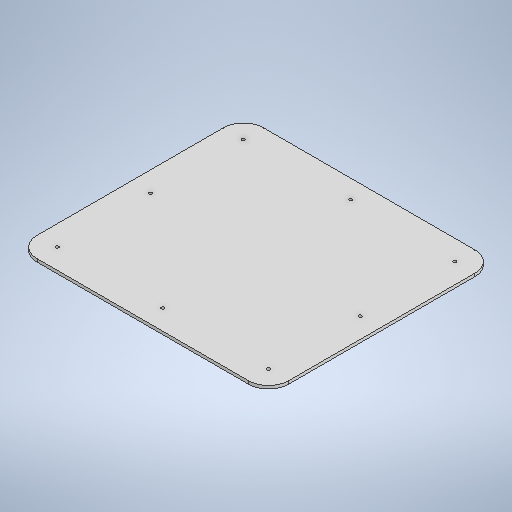
# Autodesk Inventor part: Chassis Top Plate
Saved by Autodesk Inventor 2025.2 (Build 292293000, 293)
## iProperties
Created: 2025-01-24
Part Number: Chassis Top Plate
Material: Generic
Document SubType Name: Modeling
Designer: Matt Tidd
Density: 1 g/cm^3
Appearance: Default
Author: Matt Tidd
Autodesk Inventor part; units mm, degrees
ref_plane "YZ Plane" through (0, 0, 0) normal (1, 0, 0) x (0, 1, 0)
ref_plane "XZ Plane" through (0, 0, 0) normal (0, 1, 0) x (-1, 0, 0)
ref_plane "XY Plane" through (0, 0, 0) normal (0, 0, 1) x (1, 0, 0)
sketch "Sketch2" plane through (0, 0, 0) normal (0, 1, 0) x (-1, 0, 0)
  line L0 (0, 0) -> (250, 0)
  line L1 (250, 0) -> (250, -125)
  line L2 (0, -125) -> (0, 0)
  line L3 (125, 0) -> (125, -125) construction
  line L4 (125, -125) -> (200, -125)
  line L5 (200, -125) -> (200, -225)
  line L6 (200, -225) -> (125, -225)
  line L7 (125, -225) -> (125, -125) construction
  line L8 (125, -125) -> (50, -125)
  line L9 (50, -125) -> (50, -225)
  line L10 (50, -225) -> (125, -225)
  line L11 (125, -225) -> (125, -125) construction
  line L12 (200, -125) -> (250, -125)
  line L13 (0, -125) -> (50, -125)
  line L14 (250, 0) -> (0, 0)
  line L15 (0, 0) -> (0, -225)
  line L16 (0, -225) -> (250, -225)
  line L17 (250, -225) -> (250, 0)
  dimension "d36" = 250
  dimension "d37" = 125
  dimension "d38" = 75
  dimension "d39" = 100
  dimension "d40" = 75
  dimension "d41" = 100
  constraints: 36 end point, 8 equal length, 5 horizontal, 4 perpendicular, 1 midpoint
  measures "d36" distance of L1.end L2.start
  measures "d37" distance of L0.end L1.end
  measures "d38" distance of L5.end L6.end
  measures "d39" distance of L4.end L5.end
  measures "d40" distance of L10.end L9.end
  measures "d41" distance of L9.end L8.end
extrude "Extrusion3" add sketch "Sketch2" along normal blind 3
fillet "Fillet4" radius 20 2 edges at (-250, 1.5, 0) (0, 1.5, 0)
fillet "Fillet6" radius 20 2 edges at (-250, 1.5, -225) (0, 1.5, -225)
sketch "Sketch4" plane through (0, 3, 0) normal (0, 1, 0) x (1, 0, 0)
  arc A0 (-20, 0) -> (0, 20) centre (-20, 20) ccw projected
  arc A1 (-250, 20) -> (-230, 0) centre (-230, 20) ccw projected
  arc A2 (-230, 225) -> (-250, 205) centre (-230, 205) ccw projected
  arc A3 (0, 205) -> (-20, 225) centre (-20, 205) ccw projected
  line L0 (-20, 20) -> (-20, 205) construction
  line L1 (-230, 20) -> (-230, 205) construction
  circle A4 centre (-230, 20) radius 1.5
  circle A5 centre (-20, 20) radius 1.5
  circle A6 centre (-20, 205) radius 1.5
  circle A7 centre (-230, 205) radius 1.5
  circle A8 centre (-125, 206.5) radius 1.5
  line L2 (-20, 225) -> (-230, 225) construction
  line L3 (-125, 225) -> (-125, 0) construction
  circle A9 centre (-125, 20) radius 1.5
  circle A10 centre (-230, 112.5) radius 1.5
  circle A11 centre (-20, 111) radius 1.5
  point P0 (0, 0)
  dimension "d65" = 3
  dimension "d67" = 3
  dimension "d68" = 3
  dimension "d70" = 3
  dimension "d72" = 3
  dimension "d73" = 3
  dimension "d74" = 3
  dimension "d75" = 3
  constraints: 8 centre point, 8 coincident, 6 end point, 2 midpoint, 2 point on line, 1 vertical
  measures "d65" diameter of A4
  measures "d67" diameter of A5
  measures "d68" diameter of A6
  measures "d70" diameter of A7
  measures "d72" diameter of A8
  measures "d73" diameter of A9
  measures "d74" diameter of A10
  measures "d75" diameter of A11
extrude "Extrusion5" cut sketch "Sketch4" against normal blind 3
body "Solid2"
